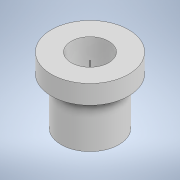
# Autodesk Inventor part: square eyelet
Saved by Autodesk Inventor 2020 (Build 240168000, 168)
## iProperties
Created: 2019-06-17
Part Number: square eyelet
Material: Generic
Document SubType Name: Modeling
Designer: ColinP
Density: 1 g/cm^3
Appearance: Default
Author: ColinP
Autodesk Inventor part; units mm, degrees
ref_plane "YZ Plane" through (0, 0, 0) normal (1, 0, 0) x (0, 1, 0)
ref_plane "XZ Plane" through (0, 0, 0) normal (0, 1, 0) x (-1, 0, 0)
ref_plane "XY Plane" through (0, 0, 0) normal (0, 0, 1) x (1, 0, 0)
sketch "Sketch1" plane through (0, 0, 0) normal (0, 1, 0) x (-1, 0, 0)
  point P0 (0, 0)
sketch "Sketch2" plane through (0, 0, 0) normal (0, 0, 1) x (1, 0, 0)
  line L0 (0, 0) -> (1.5875, 0)
  line L1 (0, 0) -> (1.5875, 0) construction
  line L2 (1.5875, 0) -> (1.5875, 5.588)
  line L3 (1.5875, 5.588) -> (0, 5.588)
  line L4 (0, 5.588) -> (3.2766, 5.588)
  line L5 (0, 0) -> (0, 3.9878)
  line L6 (0, 0) -> (3.9878, 0) construction
  line L7 (0, 3.9878) -> (3.2766, 3.9878)
  line L8 (0, 5.588) -> (0, 3.9878)
  line L9 (3.2766, 5.588) -> (3.2766, 3.9878)
  line L10 (0, 0) -> (2.4511, 0)
  line L11 (2.4511, 0) -> (2.4511, 3.9878)
  dimension "d0" = 1.5875
  dimension "d1" = 0
  dimension "d2" = 5.588
  dimension "d3" = 3.2766
  dimension "d4" = 3.9878
  dimension "d5" = 90
  dimension "d6" = 2.4511
  constraints: 24 end point, 4 horizontal, 4 perpendicular, 3 point on line, 2 equal length, 2 vertical
  measures "d0" distance of L0.start L0.end
  measures "d1" distance between parallel lines of L0 L1
  measures "d2" distance of L0.end L2.end
  measures "d3" distance of L3.end L4.end
  measures "d4" distance of L0.start L5.end
  measures "d5" angle of L6 L5
  measures "d6" distance of L0.start L10.end
sketch "Sketch3" plane through (0, 0, 0) normal (1, 0, 0) x (0, 1, 0)
  line L0 (4.9949, 0) -> (0, 0)
  constraints: 2 end point, 1 horizontal
revolve "Revolution1" add sketch "Sketch2" angle 360 about axis through (0, 5.588, 0) along (0, -1, 0) contours L2 L7 L11 L10 | L2 L4 L9 L7
body "Solid1"
